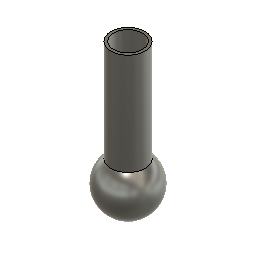
Tube (Autodesk Fusion 360 design; units mm, degrees)
part number: 2026-07-05-17-09-31-092
Autodesk Fusion 360 part; units mm, degrees
sphere "SpherePrimitive1" add diameter 80 placed x (1, 0, 0) y (0, 0, -1) z (0, 1, 0) at (0, 0, 0)
sketch "Sketch2" plane through (0, 0, 0) normal (0, 1, 0) x (1, 0, 0)
  circle A0 centre (0, 0) radius 25
  dimension "d2" = 50
  constraint coincident A0.centre origin
  measures "d2" diameter of A0
extrude "Extrude1" add sketch "Sketch2" along normal blind 200
hole "Hole1" at (0, 200, 0) direction (0, -1, 0) diameter 42 depth 170 tip angle 180
extrude "Extrude2" cut 1 faces at (23.554, 200, 1.7651) along direction (0, -1, 0) blind 20
